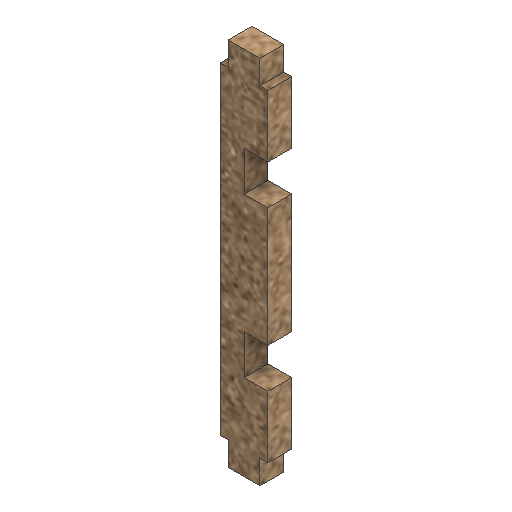
# Autodesk Inventor part: test_side_hold
Saved by Autodesk Inventor 2024 (Build 280153000, 153)
## iProperties
Created: 2024-05-27
Part Number: test_side_hold
Material: MDF Medium Density Fiberboard
Document SubType Name: Modeling
Designer: op04o
Density: 0.8 g/cm^3
Appearance: Cardboard - Corrugated
Mass: 0.57024 g
Surface Area: 8.268 cm^2
Volume: 0.7128 cm^3
Author: op04o
Autodesk Inventor part; units mm, degrees
ref_plane "YZ Plane" through (0, 0, 0) normal (1, 0, 0) x (0, 1, 0)
ref_plane "XZ Plane" through (0, 0, 0) normal (0, 1, 0) x (-1, 0, 0)
ref_plane "XY Plane" through (0, 0, 0) normal (0, 0, 1) x (1, 0, 0)
sketch "Sketch1" plane through (0, 0, 0) normal (0, 0, 1) x (1, 0, 0)
  line L0 (-3, 20.3) -> (3, 20.3)
  line L1 (3, 20.3) -> (3, -20.3)
  line L2 (3, -20.3) -> (-3, -20.3)
  line L3 (-3, -20.3) -> (-3, 20.3)
  line L4 (-2, -20.3) -> (2, -20.3)
  line L5 (2, -20.3) -> (2, -23.3)
  line L6 (2, -23.3) -> (-2, -23.3)
  line L7 (-2, -23.3) -> (-2, -20.3)
  line L8 (-2, 20.3) -> (2, 20.3)
  line L9 (2, 20.3) -> (2, 23.3)
  line L10 (2, 23.3) -> (-2, 23.3)
  line L11 (-2, 23.3) -> (-2, 20.3)
  line L12 (3, -12.5) -> (0, -12.5)
  line L13 (0, -12.5) -> (0, -7.5)
  line L14 (0, -7.5) -> (3, -7.5)
  line L15 (3, -7.5) -> (3, -12.5)
  line L16 (3, 7.5) -> (0, 7.5)
  line L17 (0, 7.5) -> (0, 12.5)
  line L18 (0, 12.5) -> (3, 12.5)
  line L19 (3, 12.5) -> (3, 7.5)
  point P0 (0, 0)
  point P1 (0, 23.3)
  point P2 (0, 20.3)
  point P3 (0, 20.3)
  point P4 (0, -23.3)
  point P5 (3, 0)
  point P6 (3, -10)
  point P7 (3, 10)
  dimension "d0" = 46.6
  dimension "d1" = 3
  dimension "d2" = 4
  dimension "d3" = 6
  dimension "d6" = 5
  dimension "d7" = 10
  dimension "d8" = 10
  dimension "d9" = 3
  constraints: 40 end point, 10 parallel, 7 midpoint, 6 point on line, 5 horizontal, 5 perpendicular, 3 vertical alignment, 2 collinear, 1 horizontal alignment
  measures "d0" distance between parallel lines of L6 L10
  measures "d1" distance of L8.end L9.end
  measures "d2" distance of L9.end L10.end
  measures "d3" distance of L0.start L0.end
  measures "d6" distance of L12.end L13.end
  measures "d7" distance of point (3, 0) point (3, -10)
  measures "d8" distance of point (3, 10) point (3, 0)
  measures "d9" distance of L13.end L14.end
extrude "Extrusion1" add sketch "Sketch1" along normal blind 3 contours L0 L1 L18 L17 L16 L14 L13 L12 L2 L3 | L11 L10 L9 L0 | L2 L5 L6 L7
body "Solid1"
